Autodesk Inventor part; units mm, degrees
(part 2 of 2)
  line L837 (-86.0406, -90.1) -> (-86.0406, -86.925)
  line L838 (-86.0406, -86.925) -> (-95.8406, -86.925)
  line L839 (-95.8406, -86.925) -> (-95.8406, -90.1)
  line L840 (-95.8406, -90.1) -> (-106.0406, -90.1)
  line L841 (-106.0406, -90.1) -> (-106.0406, -86.925)
  line L842 (-106.0406, -86.925) -> (-115.8406, -86.925)
  line L843 (-115.8406, -86.925) -> (-115.8406, -90.1)
  line L844 (-115.8406, -90.1) -> (-126.0406, -90.1)
  line L845 (-126.0406, -90.1) -> (-126.0406, -86.925)
  line L846 (-126.0406, -86.925) -> (-135.8406, -86.925)
  line L847 (-135.8406, -86.925) -> (-135.8406, -90.1)
  line L848 (-135.8406, -90.1) -> (-146.0406, -90.1)
  line L849 (-146.0406, -90.1) -> (-146.0406, -86.925)
  line L850 (-146.0406, -86.925) -> (-155.8406, -86.925)
  line L851 (-155.8406, -86.925) -> (-155.8406, -90.1)
  line L852 (-155.8406, -90.1) -> (-166.0406, -90.1)
  line L853 (-166.0406, -90.1) -> (-166.0406, -86.925)
  line L854 (-166.0406, -86.925) -> (-175.8406, -86.925)
  line L855 (-175.8406, -86.925) -> (-175.8406, -90.1)
  line L856 (-175.8406, -90.1) -> (-186.0406, -90.1)
  line L857 (-186.0406, -90.1) -> (-186.0406, -86.925)
  line L858 (-186.0406, -86.925) -> (-191.0406, -86.925)
  line L859 (-191.0406, -86.925) -> (-191.0406, -74.9)
  line L860 (-191.0406, -74.9) -> (-187.8656, -74.9)
  line L861 (-187.8656, -74.9) -> (-187.8656, -65.1)
  line L862 (-187.8656, -65.1) -> (-191.0406, -65.1)
  line L863 (-191.0406, -65.1) -> (-191.0406, -54.9)
  line L864 (-191.0406, -54.9) -> (-187.8656, -54.9)
  line L865 (-187.8656, -54.9) -> (-187.8656, -45.1)
  line L866 (-187.8656, -45.1) -> (-191.0406, -45.1)
  line L867 (-191.0406, -45.1) -> (-191.0406, -34.9)
  line L868 (-191.0406, -34.9) -> (-187.8656, -34.9)
  line L869 (-187.8656, -34.9) -> (-187.8656, -25.1)
  line L870 (-187.8656, -25.1) -> (-191.0406, -25.1)
  line L871 (-191.0406, -25.1) -> (-191.0406, -14.9)
  line L872 (-191.0406, -14.9) -> (-187.8656, -14.9)
  line L873 (-187.8656, -14.9) -> (-187.8656, -5.1)
  line L874 (-187.8656, -5.1) -> (-191.0406, -5.1)
  line L875 (-191.0406, -5.1) -> (-191.0406, 5.1)
  line L876 (-191.0406, 5.1) -> (-187.8656, 5.1)
  line L877 (-187.8656, 5.1) -> (-187.8656, 14.9)
  line L878 (-187.8656, 14.9) -> (-191.0406, 14.9)
  line L879 (-191.0406, 14.9) -> (-191.0406, 25.1)
  line L880 (-191.0406, 25.1) -> (-187.8656, 25.1)
  line L881 (-187.8656, 25.1) -> (-187.8656, 34.9)
  line L882 (-187.8656, 34.9) -> (-191.0406, 34.9)
  line L883 (-191.0406, 34.9) -> (-191.0406, 45.1)
  line L884 (-191.0406, 45.1) -> (-187.8656, 45.1)
  line L885 (-187.8656, 45.1) -> (-187.8656, 54.9)
  line L886 (-187.8656, 54.9) -> (-191.0406, 54.9)
  line L887 (-191.0406, 54.9) -> (-191.0406, 65.1)
  line L888 (-191.0406, 65.1) -> (-187.8656, 65.1)
  line L889 (-187.8656, 65.1) -> (-187.8656, 74.9)
  line L890 (-187.8656, 74.9) -> (-191.0406, 74.9)
  line L891 (-191.0406, 74.9) -> (-191.0406, 86.925)
  line L892 (-191.0406, 86.925) -> (-186.0406, 86.925)
  line L893 (-186.0406, 86.925) -> (-186.0406, 90.1)
  line L894 (-186.0406, 90.1) -> (-175.8406, 90.1)
  line L895 (-175.8406, 90.1) -> (-175.8406, 86.925)
  line L896 (-15.1, 90.1) -> (-4.9, 90.1)
  line L897 (-4.9, 90.1) -> (-4.9, 86.925)
  line L898 (-4.9, 86.925) -> (4.9, 86.925)
  line L899 (4.9, 86.925) -> (4.9, 90.1)
  line L900 (4.9, 90.1) -> (15.1, 90.1)
  line L901 (15.1, 90.1) -> (15.1, 86.925)
  line L902 (15.1, 86.925) -> (24.9, 86.925)
  line L903 (24.9, 86.925) -> (24.9, 90.1)
  line L904 (24.9, 90.1) -> (35.1, 90.1)
  line L905 (35.1, 90.1) -> (35.1, 86.925)
  line L906 (35.1, 86.925) -> (44.9, 86.925)
  line L907 (44.9, 86.925) -> (44.9, 90.1)
  line L908 (44.9, 90.1) -> (55.1, 90.1)
  line L909 (55.1, 90.1) -> (55.1, 86.925)
  line L910 (55.1, 86.925) -> (56.925, 86.925)
  line L911 (56.925, 86.925) -> (56.925, 75.1)
  line L912 (56.925, 75.1) -> (60.1, 75.1)
  line L913 (60.1, 75.1) -> (60.1, 64.9)
  line L914 (60.1, 64.9) -> (56.925, 64.9)
  line L915 (56.925, 64.9) -> (56.925, 55.1)
  line L916 (56.925, 55.1) -> (60.1, 55.1)
  line L917 (60.1, 55.1) -> (60.1, 44.9)
  line L918 (60.1, 44.9) -> (56.925, 44.9)
  line L919 (56.925, 44.9) -> (56.925, 35.1)
  line L920 (56.925, 35.1) -> (60.1, 35.1)
  line L921 (60.1, 35.1) -> (60.1, 24.9)
  line L922 (60.1, 24.9) -> (56.925, 24.9)
  line L923 (56.925, 24.9) -> (56.925, 15.1)
  line L924 (56.925, 15.1) -> (60.1, 15.1)
  line L925 (60.1, 15.1) -> (60.1, 4.9)
  line L926 (60.1, 4.9) -> (56.925, 4.9)
  line L927 (56.925, 4.9) -> (56.925, -4.9)
  line L928 (56.925, -4.9) -> (60.1, -4.9)
  line L929 (60.1, -4.9) -> (60.1, -15.1)
  line L930 (60.1, -15.1) -> (56.925, -15.1)
  line L931 (56.925, -15.1) -> (56.925, -24.9)
  line L932 (56.925, -24.9) -> (60.1, -24.9)
  line L933 (60.1, -24.9) -> (60.1, -35.1)
  line L934 (60.1, -35.1) -> (56.925, -35.1)
  line L935 (56.925, -35.1) -> (56.925, -44.9)
  line L936 (56.925, -44.9) -> (60.1, -44.9)
  line L937 (60.1, -44.9) -> (60.1, -55.1)
  line L938 (60.1, -55.1) -> (56.925, -55.1)
  line L939 (56.925, -55.1) -> (56.925, -64.9)
  line L940 (56.925, -64.9) -> (60.1, -64.9)
  line L941 (60.1, -64.9) -> (60.1, -75.1)
  line L942 (60.1, -75.1) -> (56.925, -75.1)
  line L943 (56.925, -75.1) -> (56.925, -86.925)
  line L944 (56.925, -86.925) -> (55.1, -86.925)
  line L945 (55.1, -86.925) -> (55.1, -90.1)
  line L946 (55.1, -90.1) -> (44.9, -90.1)
  line L947 (44.9, -90.1) -> (44.9, -86.925)
  line L948 (44.9, -86.925) -> (35.1, -86.925)
  line L949 (35.1, -86.925) -> (35.1, -90.1)
  line L950 (35.1, -90.1) -> (24.9, -90.1)
  line L951 (24.9, -90.1) -> (24.9, -86.925)
  line L952 (24.9, -86.925) -> (15.1, -86.925)
  line L953 (15.1, -86.925) -> (15.1, -90.1)
  line L954 (15.1, -90.1) -> (4.9, -90.1)
  line L955 (4.9, -90.1) -> (4.9, -86.925)
  line L956 (4.9, -86.925) -> (-4.9, -86.925)
  line L957 (-4.9, -86.925) -> (-4.9, -90.1)
  line L958 (-4.9, -90.1) -> (-15.1, -90.1)
  line L959 (-15.1, -90.1) -> (-15.1, -86.925)
  line L960 (-15.1, -86.925) -> (-24.9, -86.925)
  line L961 (-24.9, -86.925) -> (-24.9, -90.1)
  line L962 (-24.9, -90.1) -> (-35.1, -90.1)
  line L963 (-35.1, -90.1) -> (-35.1, -86.925)
  line L964 (-35.1, -86.925) -> (-44.9, -86.925)
  line L965 (-44.9, -86.925) -> (-44.9, -90.1)
  line L966 (-44.9, -90.1) -> (-55.1, -90.1)
  line L967 (-55.1, -90.1) -> (-55.1, -86.925)
  line L968 (-55.1, -86.925) -> (-56.925, -86.925)
  line L969 (-56.925, -86.925) -> (-56.925, -75.1)
  line L970 (-56.925, -75.1) -> (-60.1, -75.1)
  line L971 (-60.1, -75.1) -> (-60.1, -64.9)
  line L972 (-60.1, -64.9) -> (-56.925, -64.9)
  line L973 (-56.925, -64.9) -> (-56.925, -55.1)
  line L974 (-56.925, -55.1) -> (-60.1, -55.1)
  line L975 (-60.1, -55.1) -> (-60.1, -44.9)
  line L976 (-60.1, -44.9) -> (-56.925, -44.9)
  line L977 (-56.925, -44.9) -> (-56.925, -35.1)
  line L978 (-56.925, -35.1) -> (-60.1, -35.1)
  line L979 (-60.1, -35.1) -> (-60.1, -24.9)
  line L980 (-60.1, -24.9) -> (-56.925, -24.9)
  line L981 (-56.925, -24.9) -> (-56.925, -15.1)
  line L982 (-56.925, -15.1) -> (-60.1, -15.1)
  line L983 (-60.1, -15.1) -> (-60.1, -4.9)
  line L984 (-60.1, -4.9) -> (-56.925, -4.9)
  line L985 (-56.925, -4.9) -> (-56.925, 4.9)
  line L986 (-56.925, 4.9) -> (-60.1, 4.9)
  line L987 (-60.1, 4.9) -> (-60.1, 15.1)
  line L988 (-60.1, 15.1) -> (-56.925, 15.1)
  line L989 (-56.925, 15.1) -> (-56.925, 24.9)
  line L990 (-56.925, 24.9) -> (-60.1, 24.9)
  line L991 (-60.1, 24.9) -> (-60.1, 35.1)
  line L992 (-60.1, 35.1) -> (-56.925, 35.1)
  line L993 (-56.925, 35.1) -> (-56.925, 44.9)
  line L994 (-56.925, 44.9) -> (-60.1, 44.9)
  line L995 (-60.1, 44.9) -> (-60.1, 55.1)
  line L996 (-60.1, 55.1) -> (-56.925, 55.1)
  line L997 (-56.925, 55.1) -> (-56.925, 64.9)
  line L998 (-56.925, 64.9) -> (-60.1, 64.9)
  line L999 (-60.1, 64.9) -> (-60.1, 75.1)
  line L1000 (-60.1, 75.1) -> (-56.925, 75.1)
  line L1001 (-56.925, 75.1) -> (-56.925, 86.925)
  line L1002 (-56.925, 86.925) -> (-55.1, 86.925)
  line L1003 (-55.1, 86.925) -> (-55.1, 90.1)
  line L1004 (-55.1, 90.1) -> (-44.9, 90.1)
  line L1005 (-44.9, 90.1) -> (-44.9, 86.925)
  line L1006 (-44.9, 86.925) -> (-35.1, 86.925)
  line L1007 (-35.1, 86.925) -> (-35.1, 90.1)
  line L1008 (-35.1, 90.1) -> (-24.9, 90.1)
  line L1009 (-24.9, 90.1) -> (-24.9, 86.925)
  line L1010 (-24.9, 86.925) -> (-15.1, 86.925)
  line L1011 (-15.1, 86.925) -> (-15.1, 90.1)
  line L1012 (-14.9, 100.7646) -> (-25.1, 100.7646)
  line L1013 (-25.1, 100.7646) -> (-25.1, 103.9396)
  line L1014 (-25.1, 103.9396) -> (-34.9, 103.9396)
  line L1015 (-34.9, 103.9396) -> (-34.9, 100.7646)
  line L1016 (-34.9, 100.7646) -> (-45.1, 100.7646)
  line L1017 (-45.1, 100.7646) -> (-45.1, 103.9396)
  line L1018 (-45.1, 103.9396) -> (-54.9, 103.9396)
  line L1019 (-54.9, 103.9396) -> (-54.9, 100.7646)
  line L1020 (-54.9, 100.7646) -> (-60.1, 100.7646)
  line L1021 (-60.1, 100.7646) -> (-60.1, 105.9646)
  line L1022 (-60.1, 105.9646) -> (-56.925, 105.9646)
  line L1023 (-56.925, 105.9646) -> (-56.925, 115.7646)
  line L1024 (-56.925, 115.7646) -> (-60.1, 115.7646)
  line L1025 (-60.1, 115.7646) -> (-60.1, 125.9646)
  line L1026 (-60.1, 125.9646) -> (-56.925, 125.9646)
  line L1027 (-56.925, 125.9646) -> (-56.925, 135.7646)
  line L1028 (-56.925, 135.7646) -> (-60.1, 135.7646)
  line L1029 (-60.1, 135.7646) -> (-60.1, 145.9646)
  line L1030 (-60.1, 145.9646) -> (-56.925, 145.9646)
  line L1031 (-56.925, 145.9646) -> (-56.925, 155.7646)
  line L1032 (-56.925, 155.7646) -> (-60.1, 155.7646)
  line L1033 (-60.1, 155.7646) -> (-60.1, 165.9646)
  line L1034 (-60.1, 165.9646) -> (-56.925, 165.9646)
  line L1035 (-56.925, 165.9646) -> (-56.925, 175.7646)
  line L1036 (-56.925, 175.7646) -> (-60.1, 175.7646)
  line L1037 (-60.1, 175.7646) -> (-60.1, 185.9646)
  line L1038 (-60.1, 185.9646) -> (-56.925, 185.9646)
  line L1039 (-56.925, 185.9646) -> (-56.925, 195.7646)
  line L1040 (-56.925, 195.7646) -> (-60.1, 195.7646)
  line L1041 (-60.1, 195.7646) -> (-60.1, 205.9646)
  line L1042 (-60.1, 205.9646) -> (-56.925, 205.9646)
  line L1043 (-56.925, 205.9646) -> (-56.925, 215.7646)
  line L1044 (-56.925, 215.7646) -> (-60.1, 215.7646)
  line L1045 (-60.1, 215.7646) -> (-60.1, 220.9646)
  line L1046 (-60.1, 220.9646) -> (-54.9, 220.9646)
  line L1047 (-54.9, 220.9646) -> (-54.9, 217.7896)
  line L1048 (-54.9, 217.7896) -> (-45.1, 217.7896)
  line L1049 (-45.1, 217.7896) -> (-45.1, 220.9646)
  line L1050 (-45.1, 220.9646) -> (-34.9, 220.9646)
  line L1051 (-34.9, 220.9646) -> (-34.9, 217.7896)
  line L1052 (-34.9, 217.7896) -> (-25.1, 217.7896)
  line L1053 (-25.1, 217.7896) -> (-25.1, 220.9646)
  line L1054 (-25.1, 220.9646) -> (-14.9, 220.9646)
  line L1055 (-14.9, 220.9646) -> (-14.9, 217.7896)
  line L1056 (-14.9, 217.7896) -> (-5.1, 217.7896)
  line L1057 (-5.1, 217.7896) -> (-5.1, 220.9646)
  line L1058 (-5.1, 220.9646) -> (5.1, 220.9646)
  line L1059 (5.1, 220.9646) -> (5.1, 217.7896)
  line L1060 (5.1, 217.7896) -> (14.9, 217.7896)
  line L1061 (14.9, 217.7896) -> (14.9, 220.9646)
  line L1062 (14.9, 220.9646) -> (25.1, 220.9646)
  line L1063 (25.1, 220.9646) -> (25.1, 217.7896)
  line L1064 (25.1, 217.7896) -> (34.9, 217.7896)
  line L1065 (34.9, 217.7896) -> (34.9, 220.9646)
  line L1066 (34.9, 220.9646) -> (45.1, 220.9646)
  line L1067 (45.1, 220.9646) -> (45.1, 217.7896)
  line L1068 (45.1, 217.7896) -> (54.9, 217.7896)
  line L1069 (54.9, 217.7896) -> (54.9, 220.9646)
  line L1070 (54.9, 220.9646) -> (60.1, 220.9646)
  line L1071 (60.1, 220.9646) -> (60.1, 215.7646)
  line L1072 (60.1, 215.7646) -> (56.925, 215.7646)
  line L1073 (56.925, 215.7646) -> (56.925, 205.9646)
  line L1074 (56.925, 205.9646) -> (60.1, 205.9646)
  line L1075 (60.1, 205.9646) -> (60.1, 195.7646)
  line L1076 (60.1, 195.7646) -> (56.925, 195.7646)
  line L1077 (56.925, 195.7646) -> (56.925, 185.9646)
  line L1078 (56.925, 185.9646) -> (60.1, 185.9646)
  line L1079 (60.1, 185.9646) -> (60.1, 175.7646)
  line L1080 (60.1, 175.7646) -> (56.925, 175.7646)
  line L1081 (56.925, 175.7646) -> (56.925, 165.9646)
  line L1082 (56.925, 165.9646) -> (60.1, 165.9646)
  line L1083 (60.1, 165.9646) -> (60.1, 155.7646)
  line L1084 (60.1, 155.7646) -> (56.925, 155.7646)
  line L1085 (56.925, 155.7646) -> (56.925, 145.9646)
  line L1086 (56.925, 145.9646) -> (60.1, 145.9646)
  line L1087 (60.1, 145.9646) -> (60.1, 135.7646)
  line L1088 (60.1, 135.7646) -> (56.925, 135.7646)
  line L1089 (56.925, 135.7646) -> (56.925, 125.9646)
  line L1090 (56.925, 125.9646) -> (60.1, 125.9646)
  line L1091 (60.1, 125.9646) -> (60.1, 115.7646)
  line L1092 (60.1, 115.7646) -> (56.925, 115.7646)
  line L1093 (56.925, 115.7646) -> (56.925, 105.9646)
  line L1094 (56.925, 105.9646) -> (60.1, 105.9646)
  line L1095 (60.1, 105.9646) -> (60.1, 100.7646)
  line L1096 (60.1, 100.7646) -> (54.9, 100.7646)
  line L1097 (54.9, 100.7646) -> (54.9, 103.9396)
  line L1098 (54.9, 103.9396) -> (45.1, 103.9396)
  line L1099 (45.1, 103.9396) -> (45.1, 100.7646)
  line L1100 (45.1, 100.7646) -> (34.9, 100.7646)
  line L1101 (34.9, 100.7646) -> (34.9, 103.9396)
  line L1102 (34.9, 103.9396) -> (25.1, 103.9396)
  line L1103 (25.1, 103.9396) -> (25.1, 100.7646)
  line L1104 (25.1, 100.7646) -> (14.9, 100.7646)
  line L1105 (14.9, 100.7646) -> (14.9, 103.9396)
  line L1106 (14.9, 103.9396) -> (5.1, 103.9396)
  line L1107 (5.1, 103.9396) -> (5.1, 100.7646)
  line L1108 (5.1, 100.7646) -> (-5.1, 100.7646)
  line L1109 (-5.1, 100.7646) -> (-5.1, 103.9396)
  line L1110 (-5.1, 103.9396) -> (-14.9, 103.9396)
  line L1111 (-14.9, 103.9396) -> (-14.9, 100.7646)
  line L1112 (85.2973, 90.1) -> (85.2973, 86.925)
  line L1113 (85.2973, 86.925) -> (95.0973, 86.925)
  line L1114 (95.0973, 86.925) -> (95.0973, 90.1)
  line L1115 (95.0973, 90.1) -> (105.2973, 90.1)
  line L1116 (105.2973, 90.1) -> (105.2973, 86.925)
  line L1117 (105.2973, 86.925) -> (115.0973, 86.925)
  line L1118 (115.0973, 86.925) -> (115.0973, 90.1)
  line L1119 (115.0973, 90.1) -> (125.2973, 90.1)
  line L1120 (125.2973, 90.1) -> (125.2973, 86.925)
  line L1121 (125.2973, 86.925) -> (135.0973, 86.925)
  line L1122 (135.0973, 86.925) -> (135.0973, 90.1)
  line L1123 (135.0973, 90.1) -> (145.2973, 90.1)
  line L1124 (145.2973, 90.1) -> (145.2973, 86.925)
  line L1125 (145.2973, 86.925) -> (155.0973, 86.925)
  line L1126 (155.0973, 86.925) -> (155.0973, 90.1)
  line L1127 (155.0973, 90.1) -> (165.2973, 90.1)
  line L1128 (165.2973, 90.1) -> (165.2973, 86.925)
  line L1129 (165.2973, 86.925) -> (175.0973, 86.925)
  line L1130 (175.0973, 86.925) -> (175.0973, 90.1)
  line L1131 (175.0973, 90.1) -> (185.2973, 90.1)
  line L1132 (185.2973, 90.1) -> (185.2973, 86.925)
  line L1133 (185.2973, 86.925) -> (190.2973, 86.925)
  line L1134 (190.2973, 86.925) -> (190.2973, 74.9)
  line L1135 (190.2973, 74.9) -> (187.1223, 74.9)
  line L1136 (187.1223, 74.9) -> (187.1223, 65.1)
  line L1137 (187.1223, 65.1) -> (190.2973, 65.1)
  line L1138 (190.2973, 65.1) -> (190.2973, 54.9)
  line L1139 (190.2973, 54.9) -> (187.1223, 54.9)
  line L1140 (187.1223, 54.9) -> (187.1223, 45.1)
  line L1141 (187.1223, 45.1) -> (190.2973, 45.1)
  line L1142 (190.2973, 45.1) -> (190.2973, 34.9)
  line L1143 (190.2973, 34.9) -> (187.1223, 34.9)
  line L1144 (187.1223, 34.9) -> (187.1223, 25.1)
  line L1145 (187.1223, 25.1) -> (190.2973, 25.1)
  line L1146 (190.2973, 25.1) -> (190.2973, 14.9)
  line L1147 (190.2973, 14.9) -> (187.1223, 14.9)
  line L1148 (187.1223, 14.9) -> (187.1223, 5.1)
  line L1149 (187.1223, 5.1) -> (190.2973, 5.1)
  line L1150 (190.2973, 5.1) -> (190.2973, -5.1)
  line L1151 (190.2973, -5.1) -> (187.1223, -5.1)
  line L1152 (187.1223, -5.1) -> (187.1223, -14.9)
  line L1153 (187.1223, -14.9) -> (190.2973, -14.9)
  line L1154 (190.2973, -14.9) -> (190.2973, -25.1)
  line L1155 (190.2973, -25.1) -> (187.1223, -25.1)
  line L1156 (187.1223, -25.1) -> (187.1223, -34.9)
  line L1157 (187.1223, -34.9) -> (190.2973, -34.9)
  line L1158 (190.2973, -34.9) -> (190.2973, -45.1)
  line L1159 (190.2973, -45.1) -> (187.1223, -45.1)
  line L1160 (187.1223, -45.1) -> (187.1223, -54.9)
  line L1161 (187.1223, -54.9) -> (190.2973, -54.9)
  line L1162 (190.2973, -54.9) -> (190.2973, -65.1)
  line L1163 (190.2973, -65.1) -> (187.1223, -65.1)
  line L1164 (187.1223, -65.1) -> (187.1223, -74.9)
  line L1165 (187.1223, -74.9) -> (190.2973, -74.9)
  line L1166 (190.2973, -74.9) -> (190.2973, -86.925)
  line L1167 (190.2973, -86.925) -> (185.2973, -86.925)
  line L1168 (185.2973, -86.925) -> (185.2973, -90.1)
  line L1169 (185.2973, -90.1) -> (175.0973, -90.1)
  line L1170 (175.0973, -90.1) -> (175.0973, -86.925)
  line L1171 (175.0973, -86.925) -> (165.2973, -86.925)
  line L1172 (165.2973, -86.925) -> (165.2973, -90.1)
  line L1173 (165.2973, -90.1) -> (155.0973, -90.1)
  line L1174 (155.0973, -90.1) -> (155.0973, -86.925)
  line L1175 (155.0973, -86.925) -> (145.2973, -86.925)
  line L1176 (145.2973, -86.925) -> (145.2973, -90.1)
  line L1177 (145.2973, -90.1) -> (135.0973, -90.1)
  line L1178 (135.0973, -90.1) -> (135.0973, -86.925)
  line L1179 (135.0973, -86.925) -> (125.2973, -86.925)
  line L1180 (125.2973, -86.925) -> (125.2973, -90.1)
  line L1181 (125.2973, -90.1) -> (115.0973, -90.1)
  line L1182 (115.0973, -90.1) -> (115.0973, -86.925)
  line L1183 (115.0973, -86.925) -> (105.2973, -86.925)
  line L1184 (105.2973, -86.925) -> (105.2973, -90.1)
  line L1185 (105.2973, -90.1) -> (95.0973, -90.1)
  line L1186 (95.0973, -90.1) -> (95.0973, -86.925)
  line L1187 (95.0973, -86.925) -> (85.2973, -86.925)
  line L1188 (85.2973, -86.925) -> (85.2973, -90.1)
  line L1189 (85.2973, -90.1) -> (75.0973, -90.1)
  line L1190 (75.0973, -90.1) -> (75.0973, -86.925)
  line L1191 (75.0973, -86.925) -> (70.0973, -86.925)
  line L1192 (70.0973, -86.925) -> (70.0973, -74.9)
  line L1193 (70.0973, -74.9) -> (73.2723, -74.9)
  line L1194 (73.2723, -74.9) -> (73.2723, -65.1)
  line L1195 (73.2723, -65.1) -> (70.0973, -65.1)
  line L1196 (70.0973, -65.1) -> (70.0973, -54.9)
  line L1197 (70.0973, -54.9) -> (73.2723, -54.9)
  line L1198 (73.2723, -54.9) -> (73.2723, -51.4)
  line L1199 (73.2723, -51.4) -> (75.4723, -51.4)
  line L1200 (75.4723, -51.4) -> (75.4723, -52.65)
  line L1201 (75.4723, -52.65) -> (77.7723, -52.65)
  line L1202 (77.7723, -52.65) -> (77.7723, -51.4)
  line L1203 (77.7723, -51.4) -> (84.0973, -51.4)
  line L1204 (84.0973, -51.4) -> (84.0973, -48.6)
  line L1205 (84.0973, -48.6) -> (77.7723, -48.6)
  line L1206 (77.7723, -48.6) -> (77.7723, -47.35)
  line L1207 (77.7723, -47.35) -> (75.4723, -47.35)
  line L1208 (75.4723, -47.35) -> (75.4723, -48.6)
  line L1209 (75.4723, -48.6) -> (73.2723, -48.6)
  line L1210 (73.2723, -48.6) -> (73.2723, -45.1)
  line L1211 (73.2723, -45.1) -> (70.0973, -45.1)
  line L1212 (70.0973, -45.1) -> (70.0973, -34.9)
  line L1213 (70.0973, -34.9) -> (73.2723, -34.9)
  line L1214 (73.2723, -34.9) -> (73.2723, -25.1)
  line L1215 (73.2723, -25.1) -> (70.0973, -25.1)
  line L1216 (70.0973, -25.1) -> (70.0973, -14.9)
  line L1217 (70.0973, -14.9) -> (73.2723, -14.9)
  line L1218 (73.2723, -14.9) -> (73.2723, -5.1)
  line L1219 (73.2723, -5.1) -> (70.0973, -5.1)
  line L1220 (70.0973, -5.1) -> (70.0973, 5.1)
  line L1221 (70.0973, 5.1) -> (73.2723, 5.1)
  line L1222 (73.2723, 5.1) -> (73.2723, 14.9)
  line L1223 (73.2723, 14.9) -> (70.0973, 14.9)
  line L1224 (70.0973, 14.9) -> (70.0973, 25.1)
  line L1225 (70.0973, 25.1) -> (73.2723, 25.1)
  line L1226 (73.2723, 25.1) -> (73.2723, 34.9)
  line L1227 (73.2723, 34.9) -> (70.0973, 34.9)
  line L1228 (70.0973, 34.9) -> (70.0973, 45.1)
  line L1229 (70.0973, 45.1) -> (73.2723, 45.1)
  line L1230 (73.2723, 45.1) -> (73.2723, 48.6)
  line L1231 (73.2723, 48.6) -> (75.4723, 48.6)
  line L1232 (75.4723, 48.6) -> (75.4723, 47.35)
  line L1233 (75.4723, 47.35) -> (77.7723, 47.35)
  line L1234 (77.7723, 47.35) -> (77.7723, 48.6)
  line L1235 (77.7723, 48.6) -> (84.0973, 48.6)
  line L1236 (84.0973, 48.6) -> (84.0973, 51.4)
  line L1237 (84.0973, 51.4) -> (77.7723, 51.4)
  line L1238 (77.7723, 51.4) -> (77.7723, 52.65)
  line L1239 (77.7723, 52.65) -> (75.4723, 52.65)
  line L1240 (75.4723, 52.65) -> (75.4723, 51.4)
  line L1241 (75.4723, 51.4) -> (73.2723, 51.4)
  line L1242 (73.2723, 51.4) -> (73.2723, 54.9)
  line L1243 (73.2723, 54.9) -> (70.0973, 54.9)
  line L1244 (70.0973, 54.9) -> (70.0973, 65.1)
  line L1245 (70.0973, 65.1) -> (73.2723, 65.1)
  line L1246 (73.2723, 65.1) -> (73.2723, 74.9)
  line L1247 (73.2723, 74.9) -> (70.0973, 74.9)
  line L1248 (70.0973, 74.9) -> (70.0973, 86.925)
  line L1249 (70.0973, 86.925) -> (75.0973, 86.925)
  line L1250 (75.0973, 86.925) -> (75.0973, 90.1)
  line L1251 (75.0973, 90.1) -> (85.2973, 90.1)
  line L1252 (43.7, -59.9) -> (43.7, 59.9)
  line L1253 (43.7, 59.9) -> (-43.7, 59.9)
  line L1254 (-43.7, 59.9) -> (-43.7, -59.9)
  line L1255 (-43.7, -59.9) -> (43.7, -59.9)
  point P0 (0, 0)
  dimension "d8" = 0.1
  dimension "d9" = 0.1
  dimension "d10" = 0.1
  dimension "d11" = 0.1
  dimension "d12" = 0.1
  dimension "d13" = 0.1
  dimension "d14" = 0.1
  dimension "d15" = 0.1
  constraints: 1248 end point, 616 other
  measures "d8" distance between parallel lines of L8 L632
  measures "d9" distance between parallel lines of L0 L748
  measures "d10" distance between parallel lines of L6 L752
  measures "d11" distance between parallel lines of L188 L756
  measures "d12" distance between parallel lines of L377 L896
  measures "d13" distance between parallel lines of L448 L1012
  measures "d14" distance between parallel lines of L589 L1112
  measures "d15" distance between parallel lines of L268 L1252
extrude "Extrusion2" add sketch "Sketch2" along normal blind 3.175
equation "\"d8\" = laserKerf"
equation "\"d9\" = laserKerf"
equation "\"d10\" = laserKerf"
equation "\"d11\" = laserKerf"
equation "\"d12\" = laserKerf"
equation "\"d13\" = laserKerf"
equation "\"d14\" = laserKerf"
equation "\"d15\" = laserKerf"
equation "\"d16\" = materialThickness"
equation "\"materialThickness\" = 3.175"
equation "\"laserKerf\" = 0.1"
equation "\"cardPinDiameter\" = 3"
equation "\"centeralShaftDiameter\" = 8"
equation "\"cardWidth\" = 85.6"
equation "\"cardHeight\" = 53.98"
equation "\"cardThickness\" = 0.76"
equation "\"cardFillet\" = 2.88"
equation "\"cardClearence\" = 0.5"
equation "\"bearingOd\" = 22"
equation "\"bearingWidth\" = 8"
equation "\"axleHeight\" = 95"
equation "\"nutTrapClearence\" = 2"
equation "\"nutTrapwidth\" = 5.5"
equation "\"nutTrapDepth\" = 2.5"
equation "\"magnetDiameter\" = 6"
equation "\"magnetLength\" = 3"
equation "\"magnetProtusion\" = 0.25"
equation "\"spoolThickness\" = 5.588"
body "Solid2"
